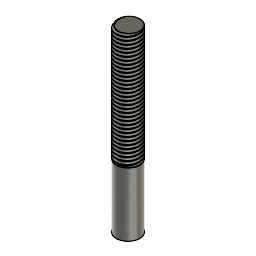
rod maker (Autodesk Fusion 360 design; units mm, degrees)
part number: 2026-06-04-10-37-24-051
Autodesk Fusion 360 part; units mm, degrees
sketch "Sketch1" plane through (0, 0, 0) normal (1, 0, 0) x (0, 1, 0)
sketch "Sketch2" plane through (0, 0, 0) normal (0, 0, 1) x (1, 0, 0)
sketch "Sketch3" plane through (0, 0, 0) normal (0, 0, 1) x (1, 0, 0)
  circle A0 centre (0, 0) radius 6
  dimension "d1" = 12
  constraint coincident A0.centre origin
  measures "d1" diameter of A0
extrude "Extrude1" add sketch "Sketch3" along normal blind 70
sketch "Sketch4" plane through (0, 0, 0) normal (1, 0, 0) x (0, 1, 0)
thread "Thread1" "ISO Metric profile 12.0 M12x1.75 M12x1.75 6g" major diameter 11.8335 minor diameter 9.8365 pitch 1.75 angle 60 modelled right hand crest width 0.2518 on face at (5.9702, -0.5974, 46.6667) from (0, 0, 12) to (0, 0, 70) crest through (5.9168, 0, -0.4375)
extrude "Extrude2" add 1 faces at (1.3581, 0.7601, 0) along direction (0, 0, -1) blind 20
named bodies: "rod maker"
